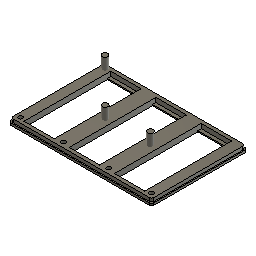
Pecon_3SlideHolder (Autodesk Fusion 360 design; units mm, degrees)
Autodesk Fusion 360 part; units mm, degrees
sketch "Sketch1" plane through (0, 0, 0) normal (0, 1, 0) x (1, 0, 0)
  line L0 (0, 0) -> (127, 0)
  line L1 (127, 0) -> (127, -85)
  line L2 (127, -85) -> (0, -85)
  line L3 (0, -85) -> (0, 0)
  line L4 (0, -42.5) -> (127, -42.5) construction
  line L5 (63.5, 0) -> (63.5, -85) construction
  line L6 (63.5, -42.5) -> (76.8, -42.5) construction
  line L7 (63.5, -42.5) -> (63.5, -4) construction
  line L8 (63.5, -4) -> (76.8, -4) construction
  line L9 (76.8, -4) -> (49.8, -4)
  line L10 (49.8, -4) -> (49.8, -81)
  line L11 (49.8, -81) -> (76.8, -81)
  line L12 (76.8, -81) -> (76.8, -4)
  line L13 (49.8, -42.5) -> (36.6, -42.5)
  line L14 (36.6, -42.5) -> (36.6, -4)
  line L15 (36.6, -4) -> (9.6, -4)
  line L16 (9.6, -4) -> (9.6, -81)
  line L17 (9.6, -81) -> (36.6, -81)
  line L18 (36.6, -81) -> (36.6, -4)
  line L19 (76.8, -42.5) -> (90, -42.5)
  line L20 (90, -42.5) -> (90, -4)
  line L21 (90, -4) -> (117, -4)
  line L22 (117, -4) -> (117, -81)
  line L23 (117, -81) -> (90, -81)
  line L24 (90, -81) -> (90, -4)
  line L25 (36.6, -42.5) -> (23.3, -42.5)
  line L26 (36.6, -4) -> (36.6, -7)
  line L27 (36.6, -7) -> (9.6, -7)
  line L28 (9.6, -7) -> (9.6, -4)
  line L29 (9.6, -4) -> (36.6, -4)
  line L30 (36.6, -4) -> (36.6, -7)
  line L31 (49.8, -4) -> (49.8, -7)
  line L32 (49.8, -7) -> (76.8, -7)
  line L33 (76.8, -7) -> (76.8, -4)
  line L34 (76.8, -4) -> (49.8, -4)
  line L35 (49.8, -4) -> (49.8, -7)
  line L36 (90, -4) -> (90, -7)
  line L37 (90, -7) -> (117, -7)
  line L38 (117, -7) -> (117, -4)
  line L39 (117, -4) -> (90, -4)
  line L40 (90, -4) -> (90, -7)
  line L41 (9.6, -81) -> (36.6, -81)
  line L42 (36.6, -81) -> (36.6, -78)
  line L43 (36.6, -78) -> (9.6, -78)
  line L44 (9.6, -78) -> (9.6, -81)
  line L45 (49.8, -81) -> (76.4, -81)
  line L46 (76.8, -78) -> (49.8, -78)
  line L47 (49.8, -78) -> (49.8, -81)
  line L48 (117, -81) -> (90.25, -81)
  line L49 (90.25, -81) -> (90.25, -78)
  line L50 (90.25, -78) -> (117, -78)
  line L51 (117, -78) -> (117, -81)
  line L52 (76.8, -42.5) -> (83.4, -42.5)
  circle A0 centre (83.4, -42.5) radius 2.5
  line L53 (36.6, -42.5) -> (43.2, -42.5)
  circle A1 centre (43.2, -42.5) radius 2.5
  line L54 (9.6, -4) -> (4.6, -4)
  circle A2 centre (4.6, -4) radius 2.5
  circle A3 centre (121.5, -79.5) radius 1.875
  circle A4 centre (83.4, -79.5) radius 1.875
  circle A5 centre (43.2, -79.5) radius 1.875
  line L55 (1, -1) -> (126, -1)
  line L56 (126, -1) -> (126, -84)
  line L57 (126, -84) -> (1, -84)
  line L58 (1, -84) -> (1, -1)
  line L59 (63.5, -1) -> (63.5, -84) construction
  line L60 (63.5, -42.5) -> (1, -42.5) construction
  line L61 (63.5, -42.5) -> (126, -42.5) construction
  line L62 (103.5, -81) -> (103.5, -4) construction
  line L63 (103.5, -42.5) -> (90, -42.5) construction
  line L64 (23.1, -81) -> (23.1, -4) construction
  circle A6 centre (5.1, -79.5) radius 1.875
  dimension "d1" = 127
  dimension "d2" = 85
  dimension "d3" = 13.3
  dimension "d4" = 38.5
  dimension "d5" = 13.3
  dimension "d6" = 27
  dimension "d8" = 13.2
  dimension "d9" = 38.5
  dimension "d10" = 27
  dimension "d12" = 13.2
  dimension "d13" = 38.5
  dimension "d14" = 27
  dimension "d15" = 77
  dimension "d16" = 13.3
  dimension "d17" = 3
  dimension "d18" = 3
  dimension "d19" = 3
  dimension "d20" = 3
  dimension "d21" = 26.6
  dimension "d22" = 3
  dimension "d23" = 3
  dimension "d42" = 6.6
  dimension "d43" = 5
  dimension "d44" = 6.6
  dimension "d45" = 5
  dimension "d50" = 5
  dimension "d51" = 5
  dimension "d63" = 3.75
  dimension "d65" = 3.75
  dimension "d67" = 3.75
  dimension "d94" = 77
  dimension "d95" = 77
  dimension "d96" = 125
  dimension "d97" = 83
  dimension "d114" = 3.75
  dimension "d116" = 4.5
  dimension "d117" = 6.6
  dimension "d118" = 6.6
  dimension "d119" = 4.5
  constraint horizontal L0
  constraint vertical L1
  constraint horizontal L2
  constraint vertical L3
  constraint coincident L0.start L3.end
  constraint midpoint L3 L4.start
  constraint midpoint L1 L4.end
  constraint midpoint L0 L5.start
  constraint midpoint L2 L5.end
  constraint midpoint L5 L6.start
  constraint coincident L4 L6.end
  constraint perpendicular L6 L7
  constraint perpendicular L5 L8
  constraint horizontal L9
  constraint vertical L10
  constraint horizontal L11
  constraint vertical L12
  constraint midpoint L10 L13.start
  constraint perpendicular L10 L13
  constraint perpendicular L4 L14
  constraint horizontal L15
  constraint vertical L16
  constraint horizontal L17
  constraint vertical L18
  constraint perpendicular L12 L19
  constraint perpendicular L19 L20
  constraint horizontal L21
  constraint vertical L22
  constraint horizontal L23
  constraint vertical L24
  constraint perpendicular L18 L25
  constraint perpendicular L15 L26
  constraint horizontal L27
  constraint vertical L28
  constraint horizontal L29
  constraint vertical L30
  constraint perpendicular L27 L31
  constraint horizontal L32
  constraint vertical L33
  constraint horizontal L34
  constraint vertical L35
  constraint perpendicular L21 L36
  constraint horizontal L37
  constraint vertical L38
  constraint horizontal L39
  constraint vertical L40
  constraint horizontal L41
  constraint vertical L42
  constraint horizontal L43
  constraint vertical L44
  constraint coincident L18 L42.end
  constraint horizontal L45
  constraint horizontal L46
  constraint vertical L47
  constraint horizontal L48
  constraint vertical L49
  constraint horizontal L50
  constraint vertical L51
  constraint perpendicular L12 L52
  constraint coincident L52.end A0.centre
  constraint perpendicular L14 L53
  constraint coincident L53.end A1.centre
  constraint perpendicular L28 L54
  constraint coincident L54.end A2.centre
  constraint horizontal L55
  constraint vertical L56
  constraint horizontal L57
  constraint vertical L58
  constraint midpoint L55 L59.start
  constraint midpoint L57 L59.end
  constraint midpoint L59 L6.start
  constraint midpoint L58 L60.end
  constraint midpoint L56 L61.end
  constraint midpoint L23 L62.start
  constraint midpoint L21 L62.end
  constraint midpoint L62 L63.start
  constraint midpoint L41 L64.start
  constraint midpoint L15 L64.end
  constraint coincident L12 L46.start
  measures "d1" distance of L0.start L0.end
  measures "d2" distance of L0.start L2.end
  measures "d3" distance of L6.start L6.end
  measures "d4" distance of L6.start L7.end
  measures "d5" distance of L7.end L8.end
  measures "d6" distance of L8.end L9.end
  measures "d8" distance of L13.start L13.end
  measures "d9" distance of L13.end L14.end
  measures "d10" distance of L14.end L15.end
  measures "d12" distance of L6.end L19.end
  measures "d13" distance of L19.end L20.end
  measures "d14" distance of L20.end L21.end
  measures "d15" distance of L20.end L23.end
  measures "d16" distance of L13.end L25.end
  measures "d17" distance of L14.end L26.end
  measures "d18" distance of L9.end L31.end
  measures "d19" distance of L20.end L36.end
  measures "d20" distance of L16.end L43.end
  measures "d21" distance of L10.end L45.end
  measures "d22" distance of L10.end L46.end
  measures "d23" distance of L22.end L50.end
  measures "d42" distance of L6.end L52.end
  measures "d43" diameter of A0
  measures "d44" distance of L13.end L53.end
  measures "d45" diameter of A1
  measures "d50" distance of L15.end L54.end
  measures "d51" diameter of A2
  measures "d63" diameter of A3
  measures "d65" diameter of A4
  measures "d67" diameter of A5
  measures "d94" distance of L9 L11
  measures "d95" distance of L15 L17
  measures "d96" distance of L55.start L55.end
  measures "d97" distance of L55.start L57.end
  measures "d114" diameter of A6
  measures "d116" distance of L22 A3.centre
  measures "d117" distance of L12 A4.centre
  measures "d118" distance of L18 A5.centre
  measures "d119" distance of L16 A6.centre
extrude "Extrude12" add sketch "Sketch1" along normal blind 15 contours A2 makes body 1
extrude "Extrude10" add sketch "Sketch1" along normal blind 15 separate body contours L13 L53 A1 | L13 L53 A1 | L19 L52 A0 | L19 L52 A0 makes body 2 at (45.6876, 10, 42.2511) makes body 3 at (85.8876, 10, 42.2511)
extrude "Extrude1" add sketch "Sketch1" along normal blind 5 separate body contours L13 L53 A1 | L13 L53 A1 | L19 L52 A0 | L19 L52 A0 | A2 | A3 | A4 | A5 | L55 L56 L57 L58 | A6 makes body 4
sketch "Sketch2" plane through (0, 5, 0) normal (0, 1, 0) x (-1, 0, 0)
  line L0 (-49.8, 81) -> (-49.8, 4)
  line L1 (-49.8, 4) -> (-76.8, 4)
  line L2 (-76.8, 4) -> (-76.8, 81)
  line L3 (-76.8, 81) -> (-49.8, 81)
  line L4 (-117, 4) -> (-117, 81)
  line L5 (-117, 81) -> (-90, 81)
  line L6 (-90, 81) -> (-90, 4)
  line L7 (-90, 4) -> (-117, 4)
  line L8 (-9.6, 81) -> (-9.6, 4)
  line L9 (-9.6, 4) -> (-36.6, 4)
  line L10 (-36.6, 4) -> (-36.6, 81)
  line L11 (-36.6, 81) -> (-9.6, 81)
  line L12 (-126, 1) -> (-1, 1)
  line L13 (-1, 1) -> (-1, 84)
  line L14 (-1, 84) -> (-126, 84)
  line L15 (-126, 84) -> (-126, 1)
  line L16 (-1.0489, 75.473) -> (-126, 75.473)
  line L17 (-126, 75.473) -> (-126, 84)
  line L18 (-126, 84) -> (-1.0489, 84)
  line L19 (-1.0489, 84) -> (-1.0489, 75.473)
  line L20 (-20.5612, 79.8702) -> (-25.5612, 79.8702)
  line L21 (-25.5612, 79.8702) -> (-25.5612, 76.8702)
  line L22 (-25.5612, 76.8702) -> (-20.5612, 76.8702)
  line L23 (-20.5612, 76.8702) -> (-20.5612, 79.8702)
  line L24 (-61.0851, 79.8702) -> (-66.0851, 79.8702)
  line L25 (-66.0851, 79.8702) -> (-66.0851, 76.8702)
  line L26 (-66.0851, 76.8702) -> (-61.0851, 76.8702)
  line L27 (-61.0851, 76.8702) -> (-61.0851, 79.8702)
  line L28 (-101.0582, 79.926) -> (-106.0582, 79.926)
  line L29 (-106.0582, 79.926) -> (-106.0582, 76.926)
  line L30 (-106.0582, 76.926) -> (-101.0582, 76.926)
  line L31 (-101.0582, 76.926) -> (-101.0582, 79.926)
  dimension "d106" = 5
  dimension "d107" = 3
  dimension "d108" = 5
  dimension "d109" = 3
  dimension "d110" = 5
  dimension "d111" = 3
  constraint horizontal L16
  constraint vertical L17
  constraint horizontal L18
  constraint vertical L19
  constraint horizontal L20
  constraint vertical L21
  constraint horizontal L22
  constraint vertical L23
  constraint horizontal L24
  constraint vertical L25
  constraint horizontal L26
  constraint vertical L27
  constraint horizontal L28
  constraint vertical L29
  constraint horizontal L30
  constraint vertical L31
  measures "d106" distance of L20.start L20.end
  measures "d107" distance of L20.start L22.end
  measures "d108" distance of L24.start L24.end
  measures "d109" distance of L24.start L26.end
  measures "d110" distance of L28.start L28.end
  measures "d111" distance of L28.start L30.end
extrude "Extrude28" add sketch "Sketch2" along normal blind 3 separate body contours L0 L2 L3 L4 L5 L6 L8 L10 L11 L14 L15 L16 L17 L18 L19 | L0 L2 L3 L16 | L8 L10 L11 L16 | L4 L5 L6 L16 | L20 L21 L22 L23 | L24 L25 L26 L27 | L28 L29 L30 L31 makes body 5
extrude "Extrude29" add sketch "Sketch2" against normal blind 4 contours L20 L21 L22 L23 | L24 L25 L26 L27 | L28 L29 L30 L31 bodies 5
extrude "Extrude4" add sketch "Sketch1" along normal blind 1 contours L9 L10 L12 L31 L32 L33 L34 L35 | L10 L11 L12 L45 L46 L47 | L14 L15 L16 L18 L26 L27 L28 L29 L30 | L16 L17 L18 L41 L42 L43 L44 | L20 L21 L22 L24 L36 L37 L38 L39 L40 | L22 L23 L48 L49 L50 L51 bodies 4
extrude "Extrude14" cut sketch "Sketch1" along normal blind 10 and the other way blind 3 contours A3 | A4 | A5 | A6 bodies 4 5
extrude "Extrude26" add sketch "Sketch1" along normal blind 2 contours L0 L1 L2 L3 bodies 4
fillet "Fillet2" radius 2 8 edges at (126, 3.5, 84) (127, 1, 85) (1, 3.5, 84) (0, 1, 85) (1, 3.5, 1) (0, 1, 0) (126, 3.5, 1) (127, 1, 0) on bodies 4
fillet "Fillet3" radius 2 3 edges at (103.5582, 1, 76.926) (63.5851, 1, 76.8702) (23.0612, 1, 76.8702) on bodies 5
fillet "Fillet4" radius 1 3 edges at (23.0612, 1, 79.8702) (63.5851, 1, 79.8702) (103.5582, 1, 79.926) on bodies 5
fillet "Fillet5" radius 1 4 edges at (1.0489, 6.5, 84) (1.0489, 6.5, 75.473) (126, 6.5, 75.473) (126, 6.5, 84) on bodies 5
hidden bodies 5
